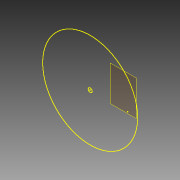
# Autodesk Inventor part: pivotMech01
Saved by Autodesk Inventor 2013 (Build 170138000, 138)
## iProperties
Created: 2013-02-19
Part Number: pivotMech01
Material: Wood (Maple)
Document SubType Name: Modeling
Designer: Nano
Mass: 275.902 g
Surface Area: 663.87 cm^2
Volume: 484.039 cm^3
Density: 0.57 g/cm^3
Author: Nano
Autodesk Inventor part; units mm, degrees
ref_plane "YZ Plane" through (0, 0, 0) normal (1, 0, 0) x (0, 1, 0)
ref_plane "XZ Plane" through (0, 0, 0) normal (0, 1, 0) x (-1, 0, 0)
ref_plane "XY Plane" through (0, 0, 0) normal (0, 0, 1) x (1, 0, 0)
ref_plane "Work Plane1" through (0, 0, -3.175) normal (0, 0, 1) x (1, 0, 0)
sketch "Sketch1" plane through (0, 0, -3.175) normal (0, 0, 1) x (1, 0, 0)
  circle A0 centre (-118.5314, 0) radius 149.2286 projected
  circle A1 centre (-118.5314, 0) radius 6.35 projected
  arc A2 (34.6158, 40.7363) -> (-271.6781, 40.7379) centre (-118.5314, 0) ccw
  line L0 (34.6158, 40.7363) -> (-271.6781, 40.7379)
  line L1 (0, 0) -> (-325.4418, 0) construction
  line L2 (34.6158, -40.7363) -> (-271.6781, -40.7379)
  arc A3 (34.6158, -40.7363) -> (34.6158, 40.7363) centre (-118.5314, 0) ccw
  arc A4 (-271.6781, 40.7379) -> (-271.6781, -40.7379) centre (-118.5314, 0) ccw
  arc A5 (-271.6781, -40.7379) -> (34.6158, -40.7363) centre (-118.5314, 0) ccw
  circle A6 centre (-187.0136, 1.9172) radius 25.6348 projected
  point P0 (0, 0)
  constraints: 8 point on circle, 6 end point, 4 centre point, 2 symmetric about line
extrude "Extrusion1" add sketch "Sketch1" along normal blind 19.05 contours A0 L2 L0 | A0 L0 A3 L2 | A0 L2 A4 L0 | A6
body "Solid1"
